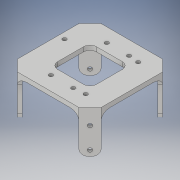
# Autodesk Inventor part: new_upper
Saved by Autodesk Inventor 2019 (Build 230136000, 136)
## iProperties
Created: 2019-02-04
Part Number: new_upper
Material: Generic
Document SubType Name: Modeling
Designer: Daniel
Density: 1 g/cm^3
Appearance: Default
Author: Daniel
Autodesk Inventor part; units mm, degrees
ref_plane "YZ Plane" through (0, 0, 0) normal (1, 0, 0) x (0, 1, 0)
ref_plane "XZ Plane" through (0, 0, 0) normal (0, 1, 0) x (-1, 0, 0)
ref_plane "XY Plane" through (0, 0, 0) normal (0, 0, 1) x (1, 0, 0)
sketch "Sketch1" plane through (0, 0, 0) normal (0, 1, 0) x (-1, 0, 0)
  line L0 (52.5, 0) -> (-52.5, 0) projected
  line L1 (0, -52.5) -> (0, 52.5) projected
  line L2 (37.5, 37.5) -> (-37.5, 37.5)
  line L3 (-37.5, 37.5) -> (-37.5, -37.5)
  line L4 (-37.5, -37.5) -> (37.5, -37.5)
  line L5 (37.5, -37.5) -> (37.5, 37.5)
  point P0 (0, 0)
  dimension "d0" = 75
  dimension "d1" = 75
  constraints: 8 end point, 2 parallel, 1 horizontal, 1 perpendicular, 2 other
  measures "d0" distance between parallel lines of L4 L2
  measures "d1" distance between parallel lines of L3 L5
extrude "Extrusion1" add sketch "Sketch1" along normal blind 4
chamfer "Chamfer2" distance 10 angle 45 4 edges at (37.5, 2, 37.5) (-37.5, 2, 37.5) (-37.5, 2, -37.5) (37.5, 2, -37.5)
sketch "Sketch11" plane through (0, 0, 0) normal (0, -1, 0) x (1, 0, 0)
  line L0 (37.5, -27.5) -> (27.5, -37.5) projected
  line L1 (37.5, 27.5) -> (37.5, -27.5) projected
  line L2 (27.5, 37.5) -> (37.5, 27.5) projected
  line L3 (-27.5, 37.5) -> (27.5, 37.5) projected
  line L4 (-37.5, 27.5) -> (-27.5, 37.5) projected
  line L5 (-37.5, -27.5) -> (-37.5, 27.5) projected
  line L6 (-27.5, -37.5) -> (-37.5, -27.5) projected
  line L7 (27.5, -37.5) -> (-27.5, -37.5) projected
  line L8 (0, -52.5) -> (0, 52.5) projected
  line L9 (-52.5, 0) -> (52.5, 0) projected
  line L10 (27.5, 37.5) -> (37.5, 27.5)
  line L11 (37.5, 27.5) -> (35.3787, 25.3787)
  line L12 (35.3787, 25.3787) -> (25.3787, 35.3787)
  line L13 (25.3787, 35.3787) -> (27.5, 37.5)
  line L14 (27.5, -37.5) -> (37.5, -27.5)
  line L15 (37.5, -27.5) -> (35.3787, -25.3787)
  line L16 (35.3787, -25.3787) -> (25.3787, -35.3787)
  line L17 (25.3787, -35.3787) -> (27.5, -37.5)
  line L18 (-37.5, -27.5) -> (-27.5, -37.5)
  line L19 (-27.5, 37.5) -> (-37.5, 27.5)
  line L20 (-37.5, 27.5) -> (-35.3787, 25.3787)
  line L21 (-35.3787, 25.3787) -> (-25.3787, 35.3787)
  line L22 (-25.3787, 35.3787) -> (-27.5, 37.5)
  line L23 (-35.3787, -25.3787) -> (-25.3787, -35.3787)
  line L24 (-37.5, -27.5) -> (-35.3787, -25.3787)
  line L25 (-25.3787, -35.3787) -> (-27.5, -37.5)
  point P0 (0, 0)
  dimension "d69" = 3
  constraints: 32 end point, 6 symmetric about line, 2 parallel, 1 perpendicular
  measures "d69" distance between parallel lines of L2 L12
extrude "Extrusion4" add sketch "Sketch11" along normal blind 34 contours L0 L17 L16 L15 | L11 L12 L13 L2 | L6 L24 L23 L25 | L22 L21 L20 L4
sketch "Sketch12" plane through (27.5, -34, 37.5) normal (0.7071068, 0, 0.7071068) x (0.7071068, 0, -0.7071068)
  line L0 (14.1421, 38) -> (0, 38) projected
  line L1 (0, 38) -> (0, 34) projected
  line L2 (0, 34) -> (0, 0) projected
  line L3 (14.1421, 0) -> (0, 0) projected
  line L4 (14.1421, 34) -> (14.1421, 0) projected
  line L5 (14.1421, 34) -> (14.1421, 38) projected
  line L6 (7.0711, 41.014) -> (7.0711, -6.6501) construction
  point P0 (7.0711, 34)
  point P1 (7.0711, 24)
  point P2 (7.0711, 5)
  dimension "d72" = 14
  dimension "d73" = 19
  constraints: 3 point on line, 2 end point, 1 vertical
  measures "d72" distance from line of L0 point (7.071, 24)
  measures "d73" distance of point (7.071, 5) point (7.071, 24)
hole "Hole4" at (32.5, -10, 32.5) at (32.5, -29, 32.5) direction (-0.7071068, 0, -0.7071068) diameter 3.5 end through all
fillet "Fillet3" radius 4 4 edges at (-30.3787, 0, -30.3787) (30.3787, 0, -30.3787) (-30.3787, 0, 30.3787) (30.3787, 0, 30.3787)
sketch "Sketch13" plane through (37.5, -34, -27.5) normal (0.7071068, 0, -0.7071068) x (-0.7071068, 0, -0.7071068)
  line L0 (14.1421, 38) -> (0, 38) projected
  line L1 (0, 38) -> (0, 34) projected
  line L2 (0, 34) -> (0, 0) projected
  line L3 (14.1421, 0) -> (0, 0) projected
  line L4 (14.1421, 34) -> (14.1421, 0) projected
  line L5 (14.1421, 34) -> (14.1421, 38) projected
  line L6 (7.0711, 44.596) -> (7.0711, -12.4532) construction
  point P0 (7.0711, 34)
  point P1 (7.0711, 24)
  point P2 (7.0711, 5)
  dimension "d82" = 14
  dimension "d83" = 19
  constraints: 3 point on line, 2 end point, 1 vertical
  measures "d82" distance from line of L0 point (7.071, 24)
  measures "d83" distance of point (7.071, 24) point (7.071, 5)
hole "Hole5" at (32.5, -10, -32.5) at (32.5, -29, -32.5) direction (-0.7071068, 0, 0.7071068) diameter 3.5 end through all
fillet "Fillet4" radius 6 8 edges at (26.4393, -34, 36.4393) (36.4393, -34, 26.4393) (26.4393, -34, -36.4393) (36.4393, -34, -26.4393) (-36.4393, -34, 26.4393) (-26.4393, -34, 36.4393) (-36.4393, -34, -26.4393) (-26.4393, -34, -36.4393)
fillet "Fillet5" radius 6 8 edges at (35.0251, 0, -25.0251) (35.0251, 0, 25.0251) (25.0251, 0, 35.0251) (-25.0251, 0, 35.0251) (-35.0251, 0, -25.0251) (-35.0251, 0, 25.0251) (25.0251, 0, -35.0251) (-25.0251, 0, -35.0251)
sketch "Sketch15" plane through (0, 0, 0) normal (0, -1, 0) x (1, 0, 0)
  line L0 (-34.3, -26.65) -> (34.3, -26.65)
  line L1 (34.3, -26.65) -> (34.3, 26.65)
  line L2 (34.3, 26.65) -> (-34.3, 26.65)
  line L3 (-34.3, 26.65) -> (-34.3, -26.65)
  line L4 (0, -52.5) -> (0, 52.5) projected
  line L5 (-52.5, 0) -> (52.5, 0) projected
  point P0 (0, 0)
  point P1 (20.3, 24.15)
  point P2 (19, -24.15)
  point P3 (-31.8, -8.95)
  dimension "d108" = 53.3
  dimension "d109" = 68.6
  dimension "d110" = 15.3
  dimension "d111" = 2.5
  dimension "d112" = 14
  dimension "d113" = 2.5
  dimension "d117" = 2.5
  dimension "d118" = 15.2
  constraints: 8 end point, 2 parallel, 1 horizontal, 1 perpendicular, 2 other
  measures "d108" distance between parallel lines of L2 L0
  measures "d109" distance between parallel lines of L1 L3
  measures "d110" distance from line of L1 point (19, -24.15)
  measures "d111" distance from line of L0 point (19, -24.15)
  measures "d112" distance from line of L1 point (20.3, 24.15)
  measures "d113" distance from line of L2 point (20.3, 24.15)
  measures "d117" distance from line of L3 point (-31.8, -8.95)
  measures "d118" vertical distance of point (19, -24.15) point (-31.8, -8.95)
hole "Hole7" at (20.3, 0, 24.15) at (19, 0, -24.15) at (-31.8, 0, -8.95) direction (0, 1, 0) diameter 3.5 end through all
sketch "Sketch16" plane through (0, 0, 0) normal (0, -1, 0) x (1, 0, 0)
  circle A0 centre (19, -24.15) radius 1.75 projected
  circle A1 centre (20.3, 24.15) radius 1.75 projected
  circle A2 centre (-31.8, -8.95) radius 1.75 projected
  line L0 (-19.0147, -37.5) -> (-18.3076, -36.7929) projected
  line L1 (19.0147, -37.5) -> (-19.0147, -37.5) projected
  line L2 (18.3076, -36.7929) -> (19.0147, -37.5) projected
  line L3 (36.7929, -18.3076) -> (18.3076, -36.7929) projected
  line L4 (37.5, -19.0147) -> (36.7929, -18.3076) projected
  line L5 (37.5, 19.0147) -> (37.5, -19.0147) projected
  line L6 (36.7929, 18.3076) -> (37.5, 19.0147) projected
  line L7 (18.3076, 36.7929) -> (36.7929, 18.3076) projected
  line L8 (19.0147, 37.5) -> (18.3076, 36.7929) projected
  line L9 (-19.0147, 37.5) -> (19.0147, 37.5) projected
  line L10 (-18.3076, 36.7929) -> (-19.0147, 37.5) projected
  line L11 (-36.7929, 18.3076) -> (-18.3076, 36.7929) projected
  line L12 (-37.5, 19.0147) -> (-36.7929, 18.3076) projected
  line L13 (-37.5, -19.0147) -> (-37.5, 19.0147) projected
  line L14 (-36.7929, -18.3076) -> (-37.5, -19.0147) projected
  line L15 (-18.3076, -36.7929) -> (-36.7929, -18.3076) projected
  line L16 (-17.5, -17.5) -> (17.5, -17.5)
  line L17 (17.5, -17.5) -> (17.5, 17.5)
  line L18 (17.5, 17.5) -> (-17.5, 17.5)
  line L19 (-17.5, 17.5) -> (-17.5, -17.5)
  line L20 (0, -52.5) -> (0, 52.5) projected
  line L21 (-52.5, 0) -> (52.5, 0) projected
  point P0 (0, 0)
  dimension "d126" = 35
  dimension "d127" = 35
  constraints: 8 end point, 2 parallel, 1 horizontal, 1 perpendicular, 2 other
  measures "d126" distance between parallel lines of L18 L16
  measures "d127" distance between parallel lines of L17 L19
extrude "Extrusion5" cut sketch "Sketch16" against normal blind 35 contours L20 L21 L17 L16 | L16 L19 L21 L20 | L21 L19 L18 L20 | L20 L18 L17 L21
fillet "Fillet6" radius 6 4 edges at (-17.5, 2, -17.5) (-17.5, 2, 17.5) (17.5, 2, -17.5) (17.5, 2, 17.5)
sketch "Sketch17" plane through (0, 0, 0) normal (0, -1, 0) x (1, 0, 0)
  line L0 (17.5, 11.5) -> (17.5, -11.5) projected
  arc A0 (11.5, -17.5) -> (17.5, -11.5) centre (11.5, -11.5) ccw projected
  line L1 (11.5, -17.5) -> (-11.5, -17.5) projected
  arc A1 (-17.5, -11.5) -> (-11.5, -17.5) centre (-11.5, -11.5) ccw projected
  line L2 (-17.5, -11.5) -> (-17.5, 11.5) projected
  arc A2 (-11.5, 17.5) -> (-17.5, 11.5) centre (-11.5, 11.5) ccw projected
  line L3 (-11.5, 17.5) -> (11.5, 17.5) projected
  arc A3 (17.5, 11.5) -> (11.5, 17.5) centre (11.5, 11.5) ccw projected
  circle A4 centre (19, -24.15) radius 1.75 projected
  circle A5 centre (20.3, 24.15) radius 1.75 projected
  circle A6 centre (-31.8, -8.95) radius 1.75 projected
  line L4 (-19.0147, -37.5) -> (-18.3076, -36.7929) projected
  line L5 (19.0147, -37.5) -> (-19.0147, -37.5) projected
  line L6 (18.3076, -36.7929) -> (19.0147, -37.5) projected
  line L7 (36.7929, -18.3076) -> (18.3076, -36.7929) projected
  line L8 (37.5, -19.0147) -> (36.7929, -18.3076) projected
  line L9 (37.5, 19.0147) -> (37.5, -19.0147) projected
  line L10 (36.7929, 18.3076) -> (37.5, 19.0147) projected
  line L11 (18.3076, 36.7929) -> (36.7929, 18.3076) projected
  line L12 (19.0147, 37.5) -> (18.3076, 36.7929) projected
  line L13 (-19.0147, 37.5) -> (19.0147, 37.5) projected
  line L14 (-18.3076, 36.7929) -> (-19.0147, 37.5) projected
  line L15 (-36.7929, 18.3076) -> (-18.3076, 36.7929) projected
  line L16 (-37.5, 19.0147) -> (-36.7929, 18.3076) projected
  line L17 (-37.5, -19.0147) -> (-37.5, 19.0147) projected
  line L18 (-36.7929, -18.3076) -> (-37.5, -19.0147) projected
  line L19 (-18.3076, -36.7929) -> (-36.7929, -18.3076) projected
  line L20 (-52.5, 0) -> (52.5, 0) projected
  line L21 (0, -52.5) -> (0, 52.5) projected
  point P0 (0, 0)
  point P1 (-10, -25)
  point P2 (10, -25)
  point P3 (-10, 25)
  point P4 (10, 25)
  dimension "d132" = 50
  dimension "d133" = 50
  dimension "d134" = 10
  dimension "d135" = 10
  constraints: 2 symmetric about line
  measures "d132" distance of point (-10, 25) point (-10, -25)
  measures "d133" distance of point (10, 25) point (10, -25)
  measures "d134" distance from line of L21 point (-10, -25)
  measures "d135" distance from line of L21 point (10, -25)
hole "Hole8" at (-10, 0, -25) at (10, 0, -25) at (-10, 0, 25) at (10, 0, 25) direction (0, 1, 0) diameter 3.5 end through all
body "Solid1"
